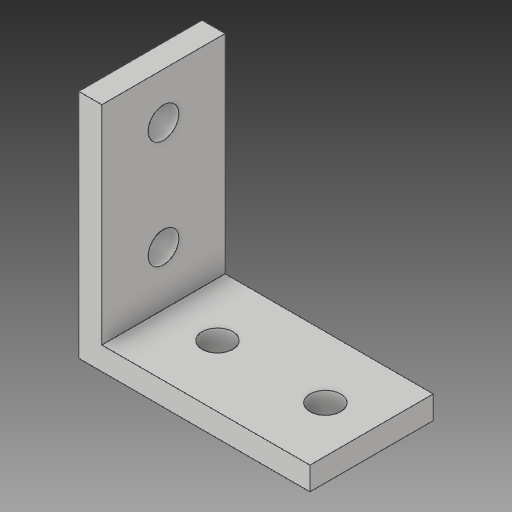
# Autodesk Inventor part: 金具 L型
Saved by Autodesk Inventor 2019 (Build 230136000, 136)
## iProperties
Created: 2020-09-29
Part Number: 金具 L型
Material: 一般
Document SubType Name: Modeling
Designer: Toshihito
Density: 1 g/cm^3
Appearance: 既定
Mass: 2.5852 g
Surface Area: 23.1227 cm^2
Volume: 2.5852 cm^3
Author: Toshihito
Autodesk Inventor part; units mm, degrees
ref_plane "YZ Plane" through (0, 0, 0) normal (1, 0, 0) x (0, 1, 0)
ref_plane "XZ Plane" through (0, 0, 0) normal (0, 1, 0) x (-1, 0, 0)
ref_plane "XY Plane" through (0, 0, 0) normal (0, 0, 1) x (1, 0, 0)
sketch "スケッチ1" plane through (0, 0, 0) normal (0, 0, 1) x (1, 0, 0)
  line L0 (0, 0) -> (3, 0)
  line L1 (3, 3) -> (3, 30)
  line L2 (3, 30) -> (0, 30)
  line L3 (0, 30) -> (0, 0)
  line L4 (0, 0) -> (30, 0)
  line L5 (30, 0) -> (30, 3)
  line L6 (30, 3) -> (3, 3)
  line L7 (0, 3) -> (0, 0)
  dimension "d0" = 3
  dimension "d1" = 30
  dimension "d2" = 30
  dimension "d3" = 3
  constraints: 16 end point, 4 parallel, 2 horizontal, 2 perpendicular
  measures "d0" distance of L2.end L1.end
  measures "d1" distance of L1.end L0.end
  measures "d2" distance of L7.start L5.end
  measures "d3" distance of L5.end L4.end
extrude "押し出し1" add sketch "スケッチ1" along normal blind 16
sketch "スケッチ2" plane through (3, 3, 0) normal (1, 0, 0) x (0, 0, -1)
  line L0 (0, 27) -> (-16, 27) construction
  line L1 (-8, 27) -> (-8, -0.1535) construction
  line L2 (-16, 27) -> (-16, -3) construction
  line L3 (-16, 7) -> (0, 7) construction
  line L4 (-16, 21) -> (-0.0153, 21) construction
  line L5 (0, 0) -> (-16, 0) construction
  point P0 (0, -3)
  point P1 (-8.0076, 21)
  point P2 (-8, 7)
  dimension "d20" = 6
  dimension "d21" = 7
  constraints: 6 end point, 3 midpoint, 2 point on line, 1 horizontal, 1 perpendicular, 1 vertical
  measures "d20" distance between parallel lines of L0 L4
  measures "d21" distance between parallel lines of L5 L3
hole "穴1" at (3, 24, 8.0076) at (3, 10, 8) direction (-1, 0, 0) diameter 4 depth 3 tip angle 118
sketch "スケッチ3" plane through (3, 3, 0) normal (0, 1, 0) x (1, 0, 0)
  line L0 (-3, -8) -> (27, -8) construction
  line L1 (27, 0) -> (27, -16) construction
  line L2 (-3, -16) -> (27, -16) construction
  line L3 (7, -16) -> (7, 0) construction
  line L4 (27, 0) -> (-3, 0) construction
  line L5 (21, -16) -> (21, 0) construction
  line L6 (0, 0) -> (0, -16) projected
  point P0 (7, -8)
  point P1 (21, -8)
  dimension "d23" = 6
  dimension "d24" = 7
  constraints: 6 end point, 3 midpoint, 2 point on line, 1 perpendicular, 1 vertical
  measures "d23" distance between parallel lines of L1 L5
  measures "d24" distance between parallel lines of L6 L3
hole "穴2" at (10, 3, 8) at (24, 3, 8) direction (0, -1, 0) diameter 4 depth 3 tip angle 118
